Autodesk Inventor part; units mm, degrees
(part 2 of 3)
sketch "Sketch13" plane through (0, 0, 3.5) normal (0, 0, 1) x (1, 0, 0)
  line L0 (21.3323, 13.0987) -> (21.3323, 4.2537) construction
  line L1 (21.3323, 4.2537) -> (17.835, 4.2537) construction
  line L2 (17.835, 4.2537) -> (17.835, 13.0987) construction
  line L3 (17.835, 13.0987) -> (21.3323, 13.0987) construction
  spline S0 degree 2 poles (20.9109, 12.1453) (20.8266, 12.1453) (20.6749, 12.2054) (20.6222, 12.2591) knots 0 0 0 1 2 2 2
  spline S1 degree 2 poles (20.6222, 12.2591) (20.5559, 12.3265) (20.4874, 12.5088) (20.4874, 12.6478) knots 0 0 0 1 2 2 2
  line L4 (20.4874, 12.6478) -> (20.4874, 12.7943)
  line L5 (20.4874, 12.7943) -> (20.0028, 12.7943)
  line L6 (20.0028, 12.7943) -> (20.0028, 12.967)
  line L7 (20.0028, 12.967) -> (21.3028, 12.967)
  line L8 (21.3028, 12.967) -> (21.3028, 12.6405)
  spline S2 degree 2 poles (21.3028, 12.6405) (21.3028, 12.5246) (21.2649, 12.3623) (21.2217, 12.3002) knots 0 0 0 1 2 2 2
  spline S3 degree 2 poles (21.2217, 12.3002) (21.1722, 12.2275) (21.0194, 12.1453) (20.9109, 12.1453) knots 0 0 0 1 2 2 2
  spline S4 degree 2 poles (20.9056, 12.3255) (20.9731, 12.3255) (21.0721, 12.3718) (21.1037, 12.4192) knots 0 0 0 1 2 2 2
  spline S5 degree 2 poles (21.1037, 12.4192) (21.1311, 12.4603) (21.1532, 12.5699) (21.1532, 12.651) knots 0 0 0 1 2 2 2
  line L9 (21.1532, 12.651) -> (21.1532, 12.7943)
  line L10 (21.1532, 12.7943) -> (20.6349, 12.7943)
  line L11 (20.6349, 12.7943) -> (20.6349, 12.6763)
  spline S6 degree 2 poles (20.6349, 12.6763) (20.6349, 12.5709) (20.6686, 12.4414) (20.7128, 12.3992) knots 0 0 0 1 2 2 2
  spline S7 degree 2 poles (20.7128, 12.3992) (20.7518, 12.3602) (20.8435, 12.3255) (20.9056, 12.3255) knots 0 0 0 1 2 2 2
  spline S8 degree 2 poles (19.9796, 11.4732) (19.9796, 11.5996) (20.0649, 11.8135) (20.1503, 11.8914) knots 0 0 0 1 2 2 2
  spline S9 degree 2 poles (20.1503, 11.8914) (20.2346, 11.9694) (20.4874, 12.0547) (20.6517, 12.0547) knots 0 0 0 1 2 2 2
  spline S10 degree 2 poles (20.6517, 12.0547) (20.815, 12.0547) (21.0573, 11.9715) (21.1469, 11.8925) knots 0 0 0 1 2 2 2
  spline S11 degree 2 poles (21.1469, 11.8925) (21.2343, 11.8145) (21.326, 11.6017) (21.326, 11.47) knots 0 0 0 1 2 2 2
  spline S12 degree 2 poles (21.326, 11.47) (21.326, 11.4047) (21.307, 11.2899) (21.2923, 11.2414) knots 0 0 0 1 2 2 2
  spline S13 degree 2 poles (21.2923, 11.2414) (21.2786, 11.1993) (21.2396, 11.1119) (21.2164, 11.0687) knots 0 0 0 1 2 2 2
  line L12 (21.2164, 11.0687) -> (21.0078, 11.0687)
  line L13 (21.0078, 11.0687) -> (21.0078, 11.0824)
  spline S14 degree 2 poles (21.0078, 11.0824) (21.0289, 11.1055) (21.0879, 11.1772) (21.1163, 11.2288) knots 0 0 0 1 2 2 2
  spline S15 degree 2 poles (21.1163, 11.2288) (21.1437, 11.2783) (21.1785, 11.3952) (21.1785, 11.4711) knots 0 0 0 1 2 2 2
  spline S16 degree 2 poles (21.1785, 11.4711) (21.1785, 11.5543) (21.11, 11.7029) (21.0447, 11.7587) knots 0 0 0 1 2 2 2
  spline S17 degree 2 poles (21.0447, 11.7587) (20.9783, 11.8135) (20.7771, 11.8746) (20.6517, 11.8746) knots 0 0 0 1 2 2 2
  spline S18 degree 2 poles (20.6517, 11.8746) (20.5179, 11.8746) (20.3252, 11.8103) (20.2588, 11.7545) knots 0 0 0 1 2 2 2
  spline S19 degree 2 poles (20.2588, 11.7545) (20.1945, 11.6997) (20.1292, 11.5533) (20.1292, 11.4711) knots 0 0 0 1 2 2 2
  spline S20 degree 2 poles (20.1292, 11.4711) (20.1292, 11.3963) (20.1661, 11.2688) (20.1935, 11.2193) knots 0 0 0 1 2 2 2
  spline S21 degree 2 poles (20.1935, 11.2193) (20.2209, 11.1719) (20.2778, 11.1013) (20.2978, 11.0813) knots 0 0 0 1 2 2 2
  line L14 (20.2978, 11.0813) -> (20.2978, 11.0687)
  line L15 (20.2978, 11.0687) -> (20.0913, 11.0687)
  spline S22 degree 2 poles (20.0913, 11.0687) (20.0713, 11.1119) (20.0344, 11.1877) (20.0175, 11.2414) knots 0 0 0 1 2 2 2
  spline S23 degree 2 poles (20.0175, 11.2414) (19.9986, 11.2983) (19.9796, 11.3952) (19.9796, 11.4732) knots 0 0 0 1 2 2 2
  line L16 (21.149, 10.13) -> (21.149, 10.7347)
  line L17 (21.149, 10.7347) -> (20.7824, 10.7347)
  line L18 (20.7824, 10.7347) -> (20.7824, 10.1553)
  line L19 (20.7824, 10.1553) -> (20.6286, 10.1553)
  line L20 (20.6286, 10.1553) -> (20.6286, 10.7347)
  line L21 (20.6286, 10.7347) -> (20.0028, 10.7347)
  line L22 (20.0028, 10.7347) -> (20.0028, 10.9075)
  line L23 (20.0028, 10.9075) -> (21.3028, 10.9075)
  line L24 (21.3028, 10.9075) -> (21.3028, 10.13)
  line L25 (21.3028, 10.13) -> (21.149, 10.13)
  spline S24 degree 2 poles (19.9733, 9.6191) (19.9733, 9.716) (20.0312, 9.8751) (20.085, 9.9309) knots 0 0 0 1 2 2 2
  spline S25 degree 2 poles (20.085, 9.9309) (20.1376, 9.9857) (20.2809, 10.0426) (20.362, 10.0426) knots 0 0 0 1 2 2 2
  spline S26 degree 2 poles (20.362, 10.0426) (20.4674, 10.0426) (20.6444, 9.9298) (20.697, 9.8224) knots 0 0 0 1 2 2 2
  line L26 (20.697, 9.8224) -> (20.7023, 9.8224)
  spline S27 degree 2 poles (20.7023, 9.8224) (20.7581, 9.9183) (20.8909, 10.011) (20.9899, 10.011) knots 0 0 0 1 2 2 2
  spline S28 degree 2 poles (20.9899, 10.011) (21.1363, 10.011) (21.3323, 9.7897) (21.3323, 9.6191) knots 0 0 0 1 2 2 2
  spline S29 degree 2 poles (21.3323, 9.6191) (21.3323, 9.4421) (21.1469, 9.2282) (21.0015, 9.2282) knots 0 0 0 1 2 2 2
  spline S30 degree 2 poles (21.0015, 9.2282) (20.9141, 9.2282) (20.7434, 9.3304) (20.6949, 9.4263) knots 0 0 0 1 2 2 2
  line L27 (20.6949, 9.4263) -> (20.6897, 9.4263)
  spline S31 degree 2 poles (20.6897, 9.4263) (20.637, 9.3125) (20.4853, 9.1956) (20.3652, 9.1956) knots 0 0 0 1 2 2 2
  spline S32 degree 2 poles (20.3652, 9.1956) (20.1987, 9.1956) (19.9733, 9.4379) (19.9733, 9.6191) knots 0 0 0 1 2 2 2
  spline S33 degree 2 poles (20.3483, 9.3747) (20.4284, 9.3747) (20.5232, 9.4379) (20.5717, 9.5274) knots 0 0 0 1 2 2 2
  spline S34 degree 2 poles (20.5717, 9.5274) (20.5885, 9.5569) (20.6275, 9.6559) (20.6528, 9.7181) knots 0 0 0 1 2 2 2
  spline S35 degree 2 poles (20.6528, 9.7181) (20.6054, 9.7897) (20.4642, 9.8666) (20.3747, 9.8666) knots 0 0 0 1 2 2 2
  spline S36 degree 2 poles (20.3747, 9.8666) (20.2567, 9.8666) (20.1029, 9.7244) (20.1029, 9.617) knots 0 0 0 1 2 2 2
  spline S37 degree 2 poles (20.1029, 9.617) (20.1029, 9.5074) (20.2346, 9.3747) (20.3483, 9.3747) knots 0 0 0 1 2 2 2
  spline S38 degree 2 poles (20.9994, 9.3989) (21.0868, 9.3989) (21.2038, 9.5158) (21.2038, 9.6201) knots 0 0 0 1 2 2 2
  spline S39 degree 2 poles (21.2038, 9.6201) (21.2038, 9.7149) (21.0995, 9.8361) (21.0099, 9.8361) knots 0 0 0 1 2 2 2
  spline S40 degree 2 poles (21.0099, 9.8361) (20.9457, 9.8361) (20.8561, 9.7739) (20.8203, 9.7118) knots 0 0 0 1 2 2 2
  spline S41 degree 2 poles (20.8203, 9.7118) (20.8055, 9.6854) (20.7539, 9.5738) (20.7392, 9.5285) knots 0 0 0 1 2 2 2
  spline S42 degree 2 poles (20.7392, 9.5285) (20.7971, 9.4526) (20.9204, 9.3989) (20.9994, 9.3989) knots 0 0 0 1 2 2 2
  spline S43 degree 2 poles (20.4158, 8.2485) (20.322, 8.2485) (20.1619, 8.3085) (20.1029, 8.3633) knots 0 0 0 1 2 2 2
  spline S44 degree 2 poles (20.1029, 8.3633) (20.0439, 8.4181) (19.9754, 8.5814) (19.9754, 8.6825) knots 0 0 0 1 2 2 2
  spline S45 degree 2 poles (19.9754, 8.6825) (19.9754, 8.7752) (20.0165, 8.9564) (20.0491, 9.0228) knots 0 0 0 1 2 2 2
  line L28 (20.0491, 9.0228) -> (20.2335, 9.0228)
  line L29 (20.2335, 9.0228) -> (20.2335, 9.0102)
  spline S46 degree 2 poles (20.2335, 9.0102) (20.2188, 8.9901) (20.1808, 8.9153) (20.164, 8.87) knots 0 0 0 1 2 2 2
  spline S47 degree 2 poles (20.164, 8.87) (20.1461, 8.8184) (20.1261, 8.7331) (20.1261, 8.6794) knots 0 0 0 1 2 2 2
  spline S48 degree 2 poles (20.1261, 8.6794) (20.1261, 8.6267) (20.164, 8.5277) (20.2051, 8.4918) knots 0 0 0 1 2 2 2
  spline S49 degree 2 poles (20.2051, 8.4918) (20.244, 8.4592) (20.3473, 8.4255) (20.4168, 8.4255) knots 0 0 0 1 2 2 2
  spline S50 degree 2 poles (20.4168, 8.4255) (20.4863, 8.4255) (20.5748, 8.4634) (20.6043, 8.4992) knots 0 0 0 1 2 2 2
  spline S51 degree 2 poles (20.6043, 8.4992) (20.637, 8.5361) (20.6644, 8.6457) (20.6644, 8.712) knots 0 0 0 1 2 2 2
  spline S52 degree 2 poles (20.6644, 8.712) (20.6644, 8.7837) (20.6423, 8.9259) (20.6328, 8.9691) knots 0 0 0 1 2 2 2
  line L30 (20.6328, 8.9691) -> (21.3028, 8.9691)
  line L31 (21.3028, 8.9691) -> (21.3028, 8.2559)
  line L32 (21.3028, 8.2559) -> (21.15, 8.2559)
  line L33 (21.15, 8.2559) -> (21.15, 8.8016)
  line L34 (21.15, 8.8016) -> (20.8034, 8.8016)
  spline S53 degree 2 poles (20.8034, 8.8016) (20.8077, 8.77) (20.8108, 8.7089) (20.8108, 8.6836) knots 0 0 0 1 2 2 2
  spline S54 degree 2 poles (20.8108, 8.6836) (20.8108, 8.5835) (20.7782, 8.4455) (20.7297, 8.3823) knots 0 0 0 1 2 2 2
  spline S55 degree 2 poles (20.7297, 8.3823) (20.6812, 8.318) (20.5337, 8.2485) (20.4158, 8.2485) knots 0 0 0 1 2 2 2
  line L35 (21.1079, 7.2445) -> (20.0028, 7.8071)
  line L36 (20.0028, 7.8071) -> (20.0028, 7.9925)
  line L37 (20.0028, 7.9925) -> (21.15, 7.3983)
  line L38 (21.15, 7.3983) -> (21.15, 8.0694)
  line L39 (21.15, 8.0694) -> (21.3028, 8.0694)
  line L40 (21.3028, 8.0694) -> (21.3028, 7.2445)
  line L41 (21.3028, 7.2445) -> (21.1079, 7.2445)
  line L42 (20.4495, 6.249) -> (20.4495, 6.4038)
  line L43 (20.4495, 6.4038) -> (20.0028, 6.4038)
  line L44 (20.0028, 6.4038) -> (20.0028, 6.5713)
  line L45 (20.0028, 6.5713) -> (20.4495, 6.5713)
  line L46 (20.4495, 6.5713) -> (20.4495, 7.1455)
  line L47 (20.4495, 7.1455) -> (20.6328, 7.1455)
  line L48 (20.6328, 7.1455) -> (21.3028, 6.564)
  line L49 (21.3028, 6.564) -> (21.3028, 6.4038)
  line L50 (21.3028, 6.4038) -> (20.5896, 6.4038)
  line L51 (20.5896, 6.4038) -> (20.5896, 6.249)
  line L52 (20.5896, 6.249) -> (20.4495, 6.249)
  line L53 (20.5896, 6.5713) -> (21.0974, 6.5713)
  line L54 (21.0974, 6.5713) -> (20.5896, 7.0085)
  line L55 (20.5896, 7.0085) -> (20.5896, 6.5713)
  line L56 (20.4495, 5.2734) -> (20.4495, 5.4283)
  line L57 (20.4495, 5.4283) -> (20.0028, 5.4283)
  line L58 (20.0028, 5.4283) -> (20.0028, 5.5958)
  line L59 (20.0028, 5.5958) -> (20.4495, 5.5958)
  line L60 (20.4495, 5.5958) -> (20.4495, 6.17)
  line L61 (20.4495, 6.17) -> (20.6328, 6.17)
  line L62 (20.6328, 6.17) -> (21.3028, 5.5884)
  line L63 (21.3028, 5.5884) -> (21.3028, 5.4283)
  line L64 (21.3028, 5.4283) -> (20.5896, 5.4283)
  line L65 (20.5896, 5.4283) -> (20.5896, 5.2734)
  line L66 (20.5896, 5.2734) -> (20.4495, 5.2734)
  line L67 (20.5896, 5.5958) -> (21.0974, 5.5958)
  line L68 (21.0974, 5.5958) -> (20.5896, 6.033)
  line L69 (20.5896, 6.033) -> (20.5896, 5.5958)
  line L70 (20.0028, 4.398) -> (20.0028, 5.0322)
  line L71 (20.0028, 5.0322) -> (20.1355, 5.0322)
  line L72 (20.1355, 5.0322) -> (20.1355, 4.7962)
  line L73 (20.1355, 4.7962) -> (21.0068, 4.7962)
  line L74 (21.0068, 4.7962) -> (21.0068, 5.0322)
  line L75 (21.0068, 5.0322) -> (21.1258, 5.0322)
  spline S56 degree 2 poles (21.1258, 5.0322) (21.1258, 4.8984) (21.2017, 4.772) (21.307, 4.7636) knots 0 0 0 1 2 2 2
  line L76 (21.307, 4.7636) -> (21.307, 4.6287)
  line L77 (21.307, 4.6287) -> (20.1355, 4.6287)
  line L78 (20.1355, 4.6287) -> (20.1355, 4.398)
  line L79 (20.1355, 4.398) -> (20.0028, 4.398)
  line L80 (17.8624, 12.0231) -> (17.8624, 12.1959)
  line L81 (17.8624, 12.1959) -> (18.4987, 12.1959)
  line L82 (18.4987, 12.1959) -> (18.4987, 12.7943)
  line L83 (18.4987, 12.7943) -> (17.8624, 12.7943)
  line L84 (17.8624, 12.7943) -> (17.8624, 12.967)
  line L85 (17.8624, 12.967) -> (19.1624, 12.967)
  line L86 (19.1624, 12.967) -> (19.1624, 12.7943)
  line L87 (19.1624, 12.7943) -> (18.6525, 12.7943)
  line L88 (18.6525, 12.7943) -> (18.6525, 12.1959)
  line L89 (18.6525, 12.1959) -> (19.1624, 12.1959)
  line L90 (19.1624, 12.1959) -> (19.1624, 12.0231)
  line L91 (19.1624, 12.0231) -> (17.8624, 12.0231)
  line L92 (17.8624, 11.0065) -> (17.8624, 11.7598)
  line L93 (17.8624, 11.7598) -> (19.1624, 11.7598)
  line L94 (19.1624, 11.7598) -> (19.1624, 11.587)
  line L95 (19.1624, 11.587) -> (18.0162, 11.587)
  line L96 (18.0162, 11.587) -> (18.0162, 11.0065)
  line L97 (18.0162, 11.0065) -> (17.8624, 11.0065)
  line L98 (19.0086, 10.0931) -> (19.0086, 10.6978)
  line L99 (19.0086, 10.6978) -> (18.642, 10.6978)
  line L100 (18.642, 10.6978) -> (18.642, 10.1184)
  line L101 (18.642, 10.1184) -> (18.4881, 10.1184)
  line L102 (18.4881, 10.1184) -> (18.4881, 10.6978)
  line L103 (18.4881, 10.6978) -> (17.8624, 10.6978)
  line L104 (17.8624, 10.6978) -> (17.8624, 10.8706)
  line L105 (17.8624, 10.8706) -> (19.1624, 10.8706)
  line L106 (19.1624, 10.8706) -> (19.1624, 10.0931)
  line L107 (19.1624, 10.0931) -> (19.0086, 10.0931)
  line L108 (17.8624, 7.4984) -> (17.8624, 8.3001)
  line L109 (17.8624, 8.3001) -> (18.0467, 8.3001)
  spline S57 degree 2 poles (18.0467, 8.3001) (18.1279, 8.2137) (18.2785, 8.0599) (18.3596, 7.9862) knots 0 0 0 1 2 2 2
  spline S58 degree 2 poles (18.3596, 7.9862) (18.5229, 7.8376) (18.7189, 7.7291) (18.8232, 7.7291) knots 0 0 0 1 2 2 2
  spline S59 degree 2 poles (18.8232, 7.7291) (18.8779, 7.7291) (18.9601, 7.7628) (18.9864, 7.7934) knots 0 0 0 1 2 2 2
  spline S60 degree 2 poles (18.9864, 7.7934) (19.0128, 7.8239) (19.0391, 7.904) (19.0391, 7.9525) knots 0 0 0 1 2 2 2
  spline S61 degree 2 poles (19.0391, 7.9525) (19.0391, 7.9988) (19.0159, 8.0936) (18.998, 8.1368) knots 0 0 0 1 2 2 2
  spline S62 degree 2 poles (18.998, 8.1368) (18.9833, 8.1737) (18.9411, 8.2422) (18.9264, 8.2632) knots 0 0 0 1 2 2 2
  line L110 (18.9264, 8.2632) -> (18.9264, 8.2727)
  line L111 (18.9264, 8.2727) -> (19.1118, 8.2727)
  spline S63 degree 2 poles (19.1118, 8.2727) (19.1381, 8.219) (19.1898, 8.0262) (19.1898, 7.9398) knots 0 0 0 1 2 2 2
  spline S64 degree 2 poles (19.1898, 7.9398) (19.1898, 7.7576) (18.997, 7.5521) (18.8326, 7.5521) knots 0 0 0 1 2 2 2
  spline S65 degree 2 poles (18.8326, 7.5521) (18.7557, 7.5521) (18.6272, 7.588) (18.5724, 7.6196) knots 0 0 0 1 2 2 2
  spline S66 degree 2 poles (18.5724, 7.6196) (18.5155, 7.6512) (18.4039, 7.7428) (18.3501, 7.7934) knots 0 0 0 1 2 2 2
  spline S67 degree 2 poles (18.3501, 7.7934) (18.2606, 7.8756) (18.0689, 8.0768) (18.013, 8.1368) knots 0 0 0 1 2 2 2
  line L112 (18.013, 8.1368) -> (18.013, 7.4984)
  line L113 (18.013, 7.4984) -> (17.8624, 7.4984)
  line L114 (17.8624, 6.5882) -> (17.8624, 7.2224)
  line L115 (17.8624, 7.2224) -> (17.9951, 7.2224)
  line L116 (17.9951, 7.2224) -> (17.9951, 6.9864)
  line L117 (17.9951, 6.9864) -> (18.8663, 6.9864)
  line L118 (18.8663, 6.9864) -> (18.8663, 7.2224)
  line L119 (18.8663, 7.2224) -> (18.9854, 7.2224)
  spline S68 degree 2 poles (18.9854, 7.2224) (18.9854, 7.0886) (19.0612, 6.9622) (19.1666, 6.9538) knots 0 0 0 1 2 2 2
  line L120 (19.1666, 6.9538) -> (19.1666, 6.8189)
  line L121 (19.1666, 6.8189) -> (17.9951, 6.8189)
  line L122 (17.9951, 6.8189) -> (17.9951, 6.5882)
  line L123 (17.9951, 6.5882) -> (17.8624, 6.5882)
  line L124 (17.8624, 6.4523) -> (19.1624, 6.014)
  line L125 (19.1624, 6.014) -> (19.1624, 5.8012)
  line L126 (19.1624, 5.8012) -> (17.8624, 5.363)
  line L127 (17.8624, 5.363) -> (17.8624, 5.5452)
  line L128 (17.8624, 5.5452) -> (18.2258, 5.6632)
  line L129 (18.2258, 5.6632) -> (18.2258, 6.1594)
  line L130 (18.2258, 6.1594) -> (17.8624, 6.2774)
  line L131 (17.8624, 6.2774) -> (17.8624, 6.4523)
  line L132 (18.3733, 5.7106) -> (18.9854, 5.9119)
  line L133 (18.9854, 5.9119) -> (18.3733, 6.112)
  line L134 (18.3733, 6.112) -> (18.3733, 5.7106)
  spline S69 degree 2 poles (18.5124, 4.4675) (18.1626, 4.4675) (17.835, 4.6709) (17.835, 4.8826) knots 0 0 0 1 2 2 2
  spline S70 degree 2 poles (17.835, 4.8826) (17.835, 5.0975) (18.1689, 5.2987) (18.5113, 5.2987) knots 0 0 0 1 2 2 2
  spline S71 degree 2 poles (18.5113, 5.2987) (18.8632, 5.2987) (19.1887, 5.0954) (19.1887, 4.8826) knots 0 0 0 1 2 2 2
  spline S72 degree 2 poles (19.1887, 4.8826) (19.1887, 4.6687) (18.8516, 4.4675) (18.5124, 4.4675) knots 0 0 0 1 2 2 2
  spline S73 degree 2 poles (18.1163, 4.6909) (18.1805, 4.6656) (18.3786, 4.6445) (18.5124, 4.6445) knots 0 0 0 1 2 2 2
  spline S74 degree 2 poles (18.5124, 4.6445) (18.6462, 4.6445) (18.8432, 4.6656) (18.9095, 4.6919) knots 0 0 0 1 2 2 2
  spline S75 degree 2 poles (18.9095, 4.6919) (18.9759, 4.7183) (19.0444, 4.8099) (19.0444, 4.8826) knots 0 0 0 1 2 2 2
  spline S76 degree 2 poles (19.0444, 4.8826) (19.0444, 4.9553) (18.9759, 5.0491) (18.9074, 5.0764) knots 0 0 0 1 2 2 2
  spline S77 degree 2 poles (18.9074, 5.0764) (18.8411, 5.1028) (18.6388, 5.1217) (18.5113, 5.1217) knots 0 0 0 1 2 2 2
  spline S78 degree 2 poles (18.5113, 5.1217) (18.3744, 5.1217) (18.1911, 5.1049) (18.1194, 5.0775) knots 0 0 0 1 2 2 2
  spline S79 degree 2 poles (18.1194, 5.0775) (18.052, 5.0522) (17.9793, 4.9585) (17.9793, 4.8826) knots 0 0 0 1 2 2 2
  spline S80 degree 2 poles (17.9793, 4.8826) (17.9793, 4.811) (18.0478, 4.7172) (18.1163, 4.6909) knots 0 0 0 1 2 2 2
  point P0 (0, 0)
  dimension "d53" = 38.1
  dimension "d54" = 0.65
  dimension "d55" = 0.65
  dimension "d56" = 0.65
  dimension "d57" = 0.65
  dimension "d58" = 2.54
  dimension "d59" = 2.54
  dimension "d60" = 2.54
  dimension "d61" = 2.54
  dimension "d62" = 2.54
  dimension "d63" = 2.54
  dimension "d64" = 2.54
  dimension "d65" = 2.54
  dimension "d66" = 2.54
  dimension "d67" = 2.54
  dimension "d68" = 2.54
  dimension "d69" = 2.54
  dimension "d70" = 2.54
  dimension "d71" = 2.54
  dimension "d100" = 1.95
  dimension "d101" = 1.95
  dimension "d102" = 1.5
  dimension "d103" = 1.5
  dimension "d104" = 19
  constraints: 2 other
extrude "Extrusion11" add sketch "Sketch13" along normal blind 0.1
sketch "Sketch15" plane through (23.35, 3.6, 1) normal (1, 0, 0) x (0, 0, -1)
  line L0 (-2, 0) -> (-2, 10.3) projected
  line L1 (0, 0) -> (-2, 0) projected
  line L2 (0, 10.3) -> (0, 0) projected
  line L3 (0, 10.3) -> (-2, 10.3) projected
  line L4 (0, 0) -> (-2, 0) projected
  line L5 (-1, 0) -> (-1, 10.3)
  line L6 (-2, 10.3) -> (-1, 10.3)
  line L7 (-2.5, 0.5) -> (-2, 0) projected
  line L8 (-2, 0) -> (-1, 0)
  line L9 (-2, 10.3) -> (-2, 0) projected
  line L10 (-1.5, 8.2889) -> (-1, 8.2889)
  line L11 (-1.5, 9.5445) -> (-1, 9.5445)
  line L12 (-1.25, 1.2556) -> (-1.25, 0.2556)
  line L13 (-1.25, 0.2556) -> (-1.75, 0.2556)
  line L14 (-1.75, 0.2556) -> (-1.75, 1.2556)
  line L15 (-1.75, 1.2556) -> (-1.25, 1.2556)
  line L16 (-1.25, 1.2556) -> (-1.75, 0.2556) construction
  line L17 (-1.25, 0.2556) -> (-1.75, 1.2556) construction
  line L18 (-1.25, 2.5111) -> (-1.25, 1.5111)
  line L19 (-1.25, 1.5111) -> (-1.75, 1.5111)
  line L20 (-1.75, 1.5111) -> (-1.75, 2.5111)
  line L21 (-1.75, 2.5111) -> (-1.25, 2.5111)
  line L22 (-1.25, 2.5111) -> (-1.75, 1.5111) construction
  line L23 (-1.25, 1.5111) -> (-1.75, 2.5111) construction
  line L24 (-1.25, 3.7667) -> (-1.25, 2.7667)
  line L25 (-1.25, 2.7667) -> (-1.75, 2.7667)
  line L26 (-1.75, 2.7667) -> (-1.75, 3.7667)
  line L27 (-1.75, 3.7667) -> (-1.25, 3.7667)
  line L28 (-1.25, 3.7667) -> (-1.75, 2.7667) construction
  line L29 (-1.25, 2.7667) -> (-1.75, 3.7667) construction
  line L30 (-1.25, 5.0222) -> (-1.25, 4.0222)
  line L31 (-1.25, 4.0222) -> (-1.75, 4.0222)
  line L32 (-1.75, 4.0222) -> (-1.75, 5.0222)
  line L33 (-1.75, 5.0222) -> (-1.25, 5.0222)
  line L34 (-1.25, 5.0222) -> (-1.75, 4.0222) construction
  line L35 (-1.25, 4.0222) -> (-1.75, 5.0222) construction
  line L36 (-1.25, 6.2778) -> (-1.25, 5.2778)
  line L37 (-1.25, 5.2778) -> (-1.75, 5.2778)
  line L38 (-1.75, 5.2778) -> (-1.75, 6.2778)
  line L39 (-1.75, 6.2778) -> (-1.25, 6.2778)
  line L40 (-1.25, 6.2778) -> (-1.75, 5.2778) construction
  line L41 (-1.25, 5.2778) -> (-1.75, 6.2778) construction
  line L42 (-1.25, 7.5334) -> (-1.25, 6.5334)
  line L43 (-1.25, 6.5334) -> (-1.75, 6.5334)
  line L44 (-1.75, 6.5334) -> (-1.75, 7.5334)
  line L45 (-1.75, 7.5334) -> (-1.25, 7.5334)
  line L46 (-1.25, 7.5334) -> (-1.75, 6.5334) construction
  line L47 (-1.25, 6.5334) -> (-1.75, 7.5334) construction
  line L48 (-1.25, 8.7889) -> (-1.25, 7.7889)
  line L49 (-1.25, 7.7889) -> (-1.75, 7.7889)
  line L50 (-1.75, 7.7889) -> (-1.75, 8.7889)
  line L51 (-1.75, 8.7889) -> (-1.25, 8.7889)
  line L52 (-1.25, 8.7889) -> (-1.75, 7.7889) construction
  line L53 (-1.25, 7.7889) -> (-1.75, 8.7889) construction
  line L54 (-1.25, 10.0445) -> (-1.25, 9.0445)
  line L55 (-1.25, 9.0445) -> (-1.75, 9.0445)
  line L56 (-1.75, 9.0445) -> (-1.75, 10.0445)
  line L57 (-1.75, 10.0445) -> (-1.25, 10.0445)
  line L58 (-1.25, 10.0445) -> (-1.75, 9.0445) construction
  line L59 (-1.25, 9.0445) -> (-1.75, 10.0445) construction
  point P0 (1, -3.6)
  dimension "d240" = 10.3
  dimension "d257" = 10.3
  dimension "d276" = 0.5
  dimension "d277" = 0.5
  dimension "d278" = 0.5
  dimension "d279" = 0.5
  dimension "d280" = 0.5
  dimension "d281" = 0.5
  dimension "d282" = 0.5
  dimension "d283" = 0.5
  constraints: 106 end point, 16 parallel, 8 perpendicular, 2 collinear, 2 horizontal, 2 midpoint
  measures "d240" distance between parallel lines of L3 L1
  measures "d257" distance of L5.start L5.end
  measures "d276" distance of L12.end L13.end
  measures "d277" distance of L19.start L19.end
  measures "d278" distance of L25.start L25.end
  measures "d279" distance of L31.start L31.end
  measures "d280" distance of L37.start L37.end
  measures "d281" distance of L43.start L43.end
  measures "d282" distance of L49.start L49.end
  measures "d283" distance of L55.start L55.end
sketch "Sketch17" plane through (16.15, 13.9, 1) normal (0, 1, 0) x (1, 0, 0)
  line L0 (7.2, -2) -> (0, -2) projected
  line L1 (7.2, 0) -> (7.2, -2) projected
  line L2 (7.2, -2) -> (7.2, 0)
  line L3 (7.2, -1) -> (7.2, -2)
  line L4 (7.2, -1.5) -> (7.45, -1.5)
  arc A0 (7.45, -1.5) -> (7.95, -1) centre (7.45, -1) ccw
  line L5 (-18.1, 0) -> (23.9, 0) projected
  line L6 (8.2, 0) -> (7.95, 0)
  arc A1 (8.45, -0.25) -> (7.95, -0.75) centre (8.45, -0.75) ccw
  line L7 (7.95, -0.75) -> (7.95, -1)
  line L8 (8.45, -0.25) -> (8.7, -0.25)
  point P0 (-16.15, 1)
  dimension "d308" = 0.25
  dimension "d309" = 0.25
  constraints: 12 end point, 4 point on circle, 2 centre point, 2 horizontal, 2 midpoint, 2 point on line, 2 vertical, 1 collinear
  measures "d308" distance of L8.start L8.end
  measures "d309" distance of L4.start L4.end
sweep "Sweep1" add profiles "Sketch15" path "Sketch17" path curves L4 A0 L7 A1 L8 contours L48 L49 L50 L51 | L54 L55 L56 L57 | L12 L13 L14 L15 | L18 L19 L20 L21 | L24 L25 L26 L27 | L30 L31 L32 L33 | L36 L37 L38 L39 | L42 L43 L44 L45
ref_plane "Work Plane1" through (19.75, 3.6, 1) normal (1, 0, 0) x (0, 0, -1)
mirror "Mirror1" about plane through (19.75, 3.6, 1) normal (1, 0, 0) of "Sweep1"
sketch "Sketch18" plane through (0, 0, 2) normal (0, 0, 1) x (1, 0, 0)
  line L0 (25.4246, 15.877) -> (25.4246, 14.777) projected
  line L1 (25.4246, 15.877) -> (23.8246, 15.877) projected
  line L2 (23.8246, 14.777) -> (23.8246, 15.877) projected
  line L3 (23.8246, 14.777) -> (25.4246, 14.777) projected
  line L4 (21.5559, 15.7398) -> (21.5559, 14.6398) projected
  line L5 (21.5559, 15.7398) -> (19.9559, 15.7398) projected
  line L6 (19.9559, 14.6398) -> (19.9559, 15.7398) projected
  line L7 (19.9559, 14.6398) -> (21.5559, 14.6398) projected
  line L8 (18.3957, 15.7376) -> (18.3957, 14.6376) projected
  line L9 (18.3957, 15.7376) -> (16.7957, 15.7376) projected
  line L10 (16.7957, 14.6376) -> (16.7957, 15.7376) projected
  line L11 (16.7957, 14.6376) -> (18.3957, 14.6376) projected
  line L12 (25.1922, 15.0759) -> (24.0666, 15.0759) construction
  line L13 (24.0666, 15.0759) -> (24.0666, 15.5865) construction
  line L14 (24.0666, 15.5865) -> (25.1922, 15.5865) construction
  line L15 (25.1922, 15.5865) -> (25.1922, 15.0759) construction
  line L16 (21.3235, 14.9388) -> (20.1979, 14.9388) construction
  line L17 (20.1979, 14.9388) -> (20.1979, 15.4493) construction
  line L18 (20.1979, 15.4493) -> (21.3235, 15.4493) construction
  line L19 (21.3235, 15.4493) -> (21.3235, 14.9388) construction
  line L20 (18.1633, 14.9366) -> (17.0377, 14.9366) construction
  line L21 (17.0377, 14.9366) -> (17.0377, 15.4471) construction
  line L22 (17.0377, 15.4471) -> (18.1633, 15.4471) construction
  line L23 (18.1633, 15.4471) -> (18.1633, 14.9366) construction
  line L24 (24.834, 15.4147) -> (24.8936, 15.4147)
  line L25 (24.8936, 15.4147) -> (24.8936, 15.5865)
  line L26 (24.8936, 15.5865) -> (24.958, 15.5865)
  line L27 (24.958, 15.5865) -> (24.958, 15.4147)
  line L28 (24.958, 15.4147) -> (25.1788, 15.4147)
  line L29 (25.1788, 15.4147) -> (25.1788, 15.3442)
  line L30 (25.1788, 15.3442) -> (24.9552, 15.0865)
  line L31 (24.9552, 15.0865) -> (24.8936, 15.0865)
  line L32 (24.8936, 15.0865) -> (24.8936, 15.3608)
  line L33 (24.8936, 15.3608) -> (24.834, 15.3608)
  line L34 (24.834, 15.3608) -> (24.834, 15.4147)
  line L35 (24.958, 15.3608) -> (24.958, 15.1655)
  line L36 (24.958, 15.1655) -> (25.1261, 15.3608)
  line L37 (25.1261, 15.3608) -> (24.958, 15.3608)
  line L38 (24.4665, 15.1614) -> (24.6829, 15.5865)
  line L39 (24.6829, 15.5865) -> (24.7542, 15.5865)
  line L40 (24.7542, 15.5865) -> (24.5257, 15.1452)
  line L41 (24.5257, 15.1452) -> (24.7838, 15.1452)
  line L42 (24.7838, 15.1452) -> (24.7838, 15.0865)
  line L43 (24.7838, 15.0865) -> (24.4665, 15.0865)
  line L44 (24.4665, 15.0865) -> (24.4665, 15.1614)
  line L45 (24.097, 15.5865) -> (24.4053, 15.5865)
  line L46 (24.4053, 15.5865) -> (24.4053, 15.5156)
  spline S0 degree 2 poles (24.4053, 15.5156) (24.3721, 15.4844) (24.3129, 15.4264) (24.2846, 15.3952) knots 0 0 0 1 2 2 2
  spline S1 degree 2 poles (24.2846, 15.3952) (24.2274, 15.3324) (24.1857, 15.2571) (24.1857, 15.2169) knots 0 0 0 1 2 2 2
  spline S2 degree 2 poles (24.1857, 15.2169) (24.1857, 15.1959) (24.1987, 15.1643) (24.2104, 15.1541) knots 0 0 0 1 2 2 2
  spline S3 degree 2 poles (24.2104, 15.1541) (24.2222, 15.144) (24.253, 15.1339) (24.2716, 15.1339) knots 0 0 0 1 2 2 2
  spline S4 degree 2 poles (24.2716, 15.1339) (24.2894, 15.1339) (24.3259, 15.1428) (24.3425, 15.1497) knots 0 0 0 1 2 2 2
  spline S5 degree 2 poles (24.3425, 15.1497) (24.3567, 15.1554) (24.383, 15.1716) (24.3911, 15.1772) knots 0 0 0 1 2 2 2
  line L47 (24.3911, 15.1772) -> (24.3948, 15.1772)
  line L48 (24.3948, 15.1772) -> (24.3948, 15.1059)
  spline S6 degree 2 poles (24.3948, 15.1059) (24.3741, 15.0958) (24.3, 15.0759) (24.2667, 15.0759) knots 0 0 0 1 2 2 2
  spline S7 degree 2 poles (24.2667, 15.0759) (24.1966, 15.0759) (24.1176, 15.1501) (24.1176, 15.2133) knots 0 0 0 1 2 2 2
  spline S8 degree 2 poles (24.1176, 15.2133) (24.1176, 15.2429) (24.1314, 15.2923) (24.1436, 15.3134) knots 0 0 0 1 2 2 2
  spline S9 degree 2 poles (24.1436, 15.3134) (24.1557, 15.3353) (24.191, 15.3782) (24.2104, 15.3989) knots 0 0 0 1 2 2 2
  spline S10 degree 2 poles (24.2104, 15.3989) (24.242, 15.4333) (24.3194, 15.5071) (24.3425, 15.5285) knots 0 0 0 1 2 2 2
  line L49 (24.3425, 15.5285) -> (24.097, 15.5285)
  line L50 (24.097, 15.5285) -> (24.097, 15.5865)
  line L51 (20.9653, 15.2775) -> (21.0249, 15.2775)
  line L52 (21.0249, 15.2775) -> (21.0249, 15.4493)
  line L53 (21.0249, 15.4493) -> (21.0893, 15.4493)
  line L54 (21.0893, 15.4493) -> (21.0893, 15.2775)
  line L55 (21.0893, 15.2775) -> (21.3101, 15.2775)
  line L56 (21.3101, 15.2775) -> (21.3101, 15.207)
  line L57 (21.3101, 15.207) -> (21.0865, 14.9493)
  line L58 (21.0865, 14.9493) -> (21.0249, 14.9493)
  line L59 (21.0249, 14.9493) -> (21.0249, 15.2236)
  line L60 (21.0249, 15.2236) -> (20.9653, 15.2236)
  line L61 (20.9653, 15.2236) -> (20.9653, 15.2775)
  line L62 (21.0893, 15.2236) -> (21.0893, 15.0283)
  line L63 (21.0893, 15.0283) -> (21.2574, 15.2236)
  line L64 (21.2574, 15.2236) -> (21.0893, 15.2236)
  line L65 (20.5978, 15.0243) -> (20.8142, 15.4493)
  line L66 (20.8142, 15.4493) -> (20.8855, 15.4493)
  line L67 (20.8855, 15.4493) -> (20.657, 15.0081)
  line L68 (20.657, 15.0081) -> (20.9151, 15.0081)
  line L69 (20.9151, 15.0081) -> (20.9151, 14.9493)
  line L70 (20.9151, 14.9493) -> (20.5978, 14.9493)
  line L71 (20.5978, 14.9493) -> (20.5978, 15.0243)
  line L72 (20.2283, 15.4493) -> (20.5366, 15.4493)
  line L73 (20.5366, 15.4493) -> (20.5366, 15.3784)
  spline S11 degree 2 poles (20.5366, 15.3784) (20.5034, 15.3472) (20.4442, 15.2893) (20.4159, 15.2581) knots 0 0 0 1 2 2 2
  spline S12 degree 2 poles (20.4159, 15.2581) (20.3587, 15.1953) (20.317, 15.1199) (20.317, 15.0798) knots 0 0 0 1 2 2 2
  spline S13 degree 2 poles (20.317, 15.0798) (20.317, 15.0587) (20.33, 15.0271) (20.3417, 15.017) knots 0 0 0 1 2 2 2
  spline S14 degree 2 poles (20.3417, 15.017) (20.3535, 15.0069) (20.3843, 14.9967) (20.4029, 14.9967) knots 0 0 0 1 2 2 2
  spline S15 degree 2 poles (20.4029, 14.9967) (20.4207, 14.9967) (20.4572, 15.0056) (20.4738, 15.0125) knots 0 0 0 1 2 2 2
  spline S16 degree 2 poles (20.4738, 15.0125) (20.488, 15.0182) (20.5143, 15.0344) (20.5224, 15.0401) knots 0 0 0 1 2 2 2
  line L74 (20.5224, 15.0401) -> (20.5261, 15.0401)
  line L75 (20.5261, 15.0401) -> (20.5261, 14.9688)
  spline S17 degree 2 poles (20.5261, 14.9688) (20.5054, 14.9586) (20.4313, 14.9388) (20.398, 14.9388) knots 0 0 0 1 2 2 2
  spline S18 degree 2 poles (20.398, 14.9388) (20.3279, 14.9388) (20.2489, 15.0129) (20.2489, 15.0761) knots 0 0 0 1 2 2 2
  spline S19 degree 2 poles (20.2489, 15.0761) (20.2489, 15.1057) (20.2627, 15.1552) (20.2749, 15.1762) knots 0 0 0 1 2 2 2
  spline S20 degree 2 poles (20.2749, 15.1762) (20.287, 15.1981) (20.3223, 15.2411) (20.3417, 15.2617) knots 0 0 0 1 2 2 2
  spline S21 degree 2 poles (20.3417, 15.2617) (20.3733, 15.2962) (20.4507, 15.3699) (20.4738, 15.3914) knots 0 0 0 1 2 2 2
  line L76 (20.4738, 15.3914) -> (20.2283, 15.3914)
  line L77 (20.2283, 15.3914) -> (20.2283, 15.4493)
  line L78 (17.8051, 15.2753) -> (17.8647, 15.2753)
  line L79 (17.8647, 15.2753) -> (17.8647, 15.4471)
  line L80 (17.8647, 15.4471) -> (17.9291, 15.4471)
  line L81 (17.9291, 15.4471) -> (17.9291, 15.2753)
  line L82 (17.9291, 15.2753) -> (18.1499, 15.2753)
  line L83 (18.1499, 15.2753) -> (18.1499, 15.2048)
  line L84 (18.1499, 15.2048) -> (17.9262, 14.9471)
  line L85 (17.9262, 14.9471) -> (17.8647, 14.9471)
  line L86 (17.8647, 14.9471) -> (17.8647, 15.2214)
  line L87 (17.8647, 15.2214) -> (17.8051, 15.2214)
  line L88 (17.8051, 15.2214) -> (17.8051, 15.2753)
  line L89 (17.9291, 15.2214) -> (17.9291, 15.0261)
  line L90 (17.9291, 15.0261) -> (18.0972, 15.2214)
  line L91 (18.0972, 15.2214) -> (17.9291, 15.2214)
  line L92 (17.4376, 15.0221) -> (17.654, 15.4471)
  line L93 (17.654, 15.4471) -> (17.7253, 15.4471)
  line L94 (17.7253, 15.4471) -> (17.4967, 15.0059)
  line L95 (17.4967, 15.0059) -> (17.7549, 15.0059)
  line L96 (17.7549, 15.0059) -> (17.7549, 14.9471)
  line L97 (17.7549, 14.9471) -> (17.4376, 14.9471)
  line L98 (17.4376, 14.9471) -> (17.4376, 15.0221)
  line L99 (17.0681, 15.4471) -> (17.3764, 15.4471)
  line L100 (17.3764, 15.4471) -> (17.3764, 15.3762)
  spline S22 degree 2 poles (17.3764, 15.3762) (17.3432, 15.345) (17.284, 15.2871) (17.2557, 15.2559) knots 0 0 0 1 2 2 2
  spline S23 degree 2 poles (17.2557, 15.2559) (17.1985, 15.1931) (17.1568, 15.1177) (17.1568, 15.0776) knots 0 0 0 1 2 2 2
  spline S24 degree 2 poles (17.1568, 15.0776) (17.1568, 15.0565) (17.1698, 15.0249) (17.1815, 15.0148) knots 0 0 0 1 2 2 2
  spline S25 degree 2 poles (17.1815, 15.0148) (17.1933, 15.0046) (17.2241, 14.9945) (17.2427, 14.9945) knots 0 0 0 1 2 2 2
  spline S26 degree 2 poles (17.2427, 14.9945) (17.2605, 14.9945) (17.297, 15.0034) (17.3136, 15.0103) knots 0 0 0 1 2 2 2
  spline S27 degree 2 poles (17.3136, 15.0103) (17.3278, 15.016) (17.3541, 15.0322) (17.3622, 15.0379) knots 0 0 0 1 2 2 2
  line L101 (17.3622, 15.0379) -> (17.3659, 15.0379)
  line L102 (17.3659, 15.0379) -> (17.3659, 14.9666)
  spline S28 degree 2 poles (17.3659, 14.9666) (17.3452, 14.9564) (17.2711, 14.9366) (17.2378, 14.9366) knots 0 0 0 1 2 2 2
  spline S29 degree 2 poles (17.2378, 14.9366) (17.1677, 14.9366) (17.0887, 15.0107) (17.0887, 15.0739) knots 0 0 0 1 2 2 2
  spline S30 degree 2 poles (17.0887, 15.0739) (17.0887, 15.1035) (17.1025, 15.1529) (17.1147, 15.174) knots 0 0 0 1 2 2 2
  spline S31 degree 2 poles (17.1147, 15.174) (17.1268, 15.1959) (17.1621, 15.2388) (17.1815, 15.2595) knots 0 0 0 1 2 2 2
  spline S32 degree 2 poles (17.1815, 15.2595) (17.2131, 15.294) (17.2905, 15.3677) (17.3136, 15.3892) knots 0 0 0 1 2 2 2
  line L103 (17.3136, 15.3892) -> (17.0681, 15.3892)
  line L104 (17.0681, 15.3892) -> (17.0681, 15.4471)
  point P0 (0, 0)
  dimension "d53" = 38.1
  dimension "d54" = 0.65
  dimension "d55" = 0.65
  dimension "d56" = 0.65
  dimension "d57" = 0.65
  dimension "d58" = 2.54
  dimension "d59" = 2.54
  dimension "d60" = 2.54
  dimension "d61" = 2.54
  dimension "d62" = 2.54
  dimension "d63" = 2.54
  dimension "d64" = 2.54
  dimension "d65" = 2.54
  dimension "d66" = 2.54
  dimension "d67" = 2.54
  dimension "d68" = 2.54
  dimension "d69" = 2.54
  dimension "d70" = 2.54
  dimension "d71" = 2.54
  dimension "d100" = 1.95
  dimension "d101" = 1.95
  dimension "d102" = 1.5
  dimension "d103" = 1.5
  dimension "d104" = 19
  constraints: 6 other
extrude "Extrusion12" add sketch "Sketch18" along normal blind 0.1 contours L24 L25 L26 L27 L28 L29 L30 L31 L32 L33 L34 | L38 L39 L40 L41 L42 L43 L44 | L45 L46 S0 S1 S2 S3 S4 S5 L47 L48 S6 S7 S8 S9 S10 L49 L50 | L51 L52 L53 L54 L55 L56 L57 L58 L59 L60 L61 | L65 L66 L67 L68 L69 L70 L71 | L72 L73 S11 S12 S13 S14 S15 S16 L74 L75 S17 S18 S19 S20 S21 L76 L77 | L78 L79 L80 L81 L82 L83 L84 L85 L86 L87 L88 | L92 L93 L94 L95 L96 L97 L98 | L99 L100 S22 S23 S24 S25 S26 S27 L101 L102 S28 S29 S30 S31 S32 L103 L104
sketch "Sketch19" plane through (0, 0, 2) normal (0, 0, 1) x (1, 0, 0)
  line L0 (28.2585, 12.9872) -> (29.3585, 12.9872) projected
  line L1 (28.2585, 12.9872) -> (28.2585, 11.3872) projected
  line L2 (29.3585, 11.3872) -> (28.2585, 11.3872) projected
  line L3 (29.3585, 11.3872) -> (29.3585, 12.9872) projected
  line L4 (31.1887, 11.3872) -> (30.0887, 11.3872) projected
  line L5 (31.1887, 11.3872) -> (31.1887, 12.9872) projected
  line L6 (30.0887, 12.9872) -> (31.1887, 12.9872) projected
  line L7 (30.0887, 12.9872) -> (30.0887, 11.3872) projected
  line L8 (31.8382, 12.9872) -> (32.9382, 12.9872) projected
  line L9 (31.8382, 12.9872) -> (31.8382, 11.3872) projected
  line L10 (32.9382, 11.3872) -> (31.8382, 11.3872) projected
  line L11 (32.9382, 11.3872) -> (32.9382, 12.9872) projected
  line L12 (28.495, 11.6041) -> (28.495, 13.8553) construction
  line L13 (28.495, 13.8553) -> (29.516, 13.8553) construction
  line L14 (29.516, 13.8553) -> (29.516, 11.6041) construction
  line L15 (29.516, 11.6041) -> (28.495, 11.6041) construction
  line L16 (30.3322, 11.6041) -> (30.3322, 13.8553) construction
  line L17 (30.3322, 13.8553) -> (31.3533, 13.8553) construction
  line L18 (31.3533, 13.8553) -> (31.3533, 11.6041) construction
  line L19 (31.3533, 11.6041) -> (30.3322, 11.6041) construction
  line L20 (32.1266, 11.6413) -> (32.1266, 12.7669) construction
  line L21 (32.1266, 12.7669) -> (32.6476, 12.7669) construction
  line L22 (32.6476, 12.7669) -> (32.6476, 11.6413) construction
  line L23 (32.6476, 11.6413) -> (32.1266, 11.6413) construction
  line L24 (32.6371, 11.961) -> (32.6371, 11.7171)
  line L25 (32.6371, 11.7171) -> (32.586, 11.7171)
  line L26 (32.586, 11.7171) -> (32.586, 11.8078)
  line L27 (32.586, 11.8078) -> (32.2509, 11.8078)
  line L28 (32.2509, 11.8078) -> (32.2509, 11.7171)
  line L29 (32.2509, 11.7171) -> (32.2052, 11.7171)
  spline S0 degree 2 poles (32.2052, 11.7171) (32.2052, 11.7685) (32.176, 11.8171) (32.1355, 11.8204) knots 0 0 0 1 2 2 2
  line L30 (32.1355, 11.8204) -> (32.1355, 11.8722)
  line L31 (32.1355, 11.8722) -> (32.586, 11.8722)
  line L32 (32.586, 11.8722) -> (32.586, 11.961)
  line L33 (32.586, 11.961) -> (32.6371, 11.961)
  spline S1 degree 2 poles (32.3871, 12.3641) (32.5216, 12.3641) (32.6476, 12.2859) (32.6476, 12.2045) knots 0 0 0 1 2 2 2
  spline S2 degree 2 poles (32.6476, 12.2045) (32.6476, 12.1218) (32.5192, 12.0444) (32.3875, 12.0444) knots 0 0 0 1 2 2 2
  spline S3 degree 2 poles (32.3875, 12.0444) (32.2522, 12.0444) (32.127, 12.1226) (32.127, 12.2045) knots 0 0 0 1 2 2 2
  spline S4 degree 2 poles (32.127, 12.2045) (32.127, 12.2867) (32.2566, 12.3641) (32.3871, 12.3641) knots 0 0 0 1 2 2 2
  spline S5 degree 2 poles (32.5394, 12.2782) (32.5147, 12.288) (32.4385, 12.2961) (32.3871, 12.2961) knots 0 0 0 1 2 2 2
  spline S6 degree 2 poles (32.3871, 12.2961) (32.3356, 12.2961) (32.2599, 12.288) (32.2343, 12.2778) knots 0 0 0 1 2 2 2
  spline S7 degree 2 poles (32.2343, 12.2778) (32.2088, 12.2677) (32.1825, 12.2324) (32.1825, 12.2045) knots 0 0 0 1 2 2 2
  spline S8 degree 2 poles (32.1825, 12.2045) (32.1825, 12.1765) (32.2088, 12.1405) (32.2351, 12.1299) knots 0 0 0 1 2 2 2
  spline S9 degree 2 poles (32.2351, 12.1299) (32.2607, 12.1198) (32.3385, 12.1125) (32.3875, 12.1125) knots 0 0 0 1 2 2 2
  spline S10 degree 2 poles (32.3875, 12.1125) (32.4402, 12.1125) (32.5107, 12.119) (32.5382, 12.1295) knots 0 0 0 1 2 2 2
  spline S11 degree 2 poles (32.5382, 12.1295) (32.5642, 12.1393) (32.5921, 12.1753) (32.5921, 12.2045) knots 0 0 0 1 2 2 2
  spline S12 degree 2 poles (32.5921, 12.2045) (32.5921, 12.232) (32.5658, 12.2681) (32.5394, 12.2782) knots 0 0 0 1 2 2 2
  line L34 (32.6371, 12.7365) -> (32.6371, 12.4282)
  line L35 (32.6371, 12.4282) -> (32.5662, 12.4282)
  spline S13 degree 2 poles (32.5662, 12.4282) (32.535, 12.4614) (32.477, 12.5205) (32.4458, 12.5489) knots 0 0 0 1 2 2 2
  spline S14 degree 2 poles (32.4458, 12.5489) (32.383, 12.606) (32.3077, 12.6478) (32.2676, 12.6478) knots 0 0 0 1 2 2 2
  spline S15 degree 2 poles (32.2676, 12.6478) (32.2465, 12.6478) (32.2149, 12.6348) (32.2048, 12.623) knots 0 0 0 1 2 2 2
  spline S16 degree 2 poles (32.2048, 12.623) (32.1946, 12.6113) (32.1845, 12.5805) (32.1845, 12.5619) knots 0 0 0 1 2 2 2
  spline S17 degree 2 poles (32.1845, 12.5619) (32.1845, 12.544) (32.1934, 12.5076) (32.2003, 12.491) knots 0 0 0 1 2 2 2
  spline S18 degree 2 poles (32.2003, 12.491) (32.206, 12.4768) (32.2222, 12.4504) (32.2279, 12.4423) knots 0 0 0 1 2 2 2
  line L36 (32.2279, 12.4423) -> (32.2279, 12.4387)
  line L37 (32.2279, 12.4387) -> (32.1565, 12.4387)
  spline S19 degree 2 poles (32.1565, 12.4387) (32.1464, 12.4594) (32.1266, 12.5335) (32.1266, 12.5667) knots 0 0 0 1 2 2 2
  spline S20 degree 2 poles (32.1266, 12.5667) (32.1266, 12.6368) (32.2007, 12.7158) (32.2639, 12.7158) knots 0 0 0 1 2 2 2
  spline S21 degree 2 poles (32.2639, 12.7158) (32.2935, 12.7158) (32.3429, 12.7021) (32.364, 12.6899) knots 0 0 0 1 2 2 2
  spline S22 degree 2 poles (32.364, 12.6899) (32.3859, 12.6777) (32.4288, 12.6425) (32.4495, 12.623) knots 0 0 0 1 2 2 2
  spline S23 degree 2 poles (32.4495, 12.623) (32.4839, 12.5914) (32.5577, 12.5141) (32.5791, 12.491) knots 0 0 0 1 2 2 2
  line L38 (32.5791, 12.491) -> (32.5791, 12.7365)
  line L39 (32.5791, 12.7365) -> (32.6371, 12.7365)
  line L40 (30.6709, 11.9622) -> (30.6709, 11.9027)
  line L41 (30.6709, 11.9027) -> (30.8427, 11.9027)
  line L42 (30.8427, 11.9027) -> (30.8427, 11.8383)
  line L43 (30.8427, 11.8383) -> (30.6709, 11.8383)
  line L44 (30.6709, 11.8383) -> (30.6709, 11.6174)
  line L45 (30.6709, 11.6174) -> (30.6004, 11.6174)
  line L46 (30.6004, 11.6174) -> (30.3427, 11.8411)
  line L47 (30.3427, 11.8411) -> (30.3427, 11.9027)
  line L48 (30.3427, 11.9027) -> (30.617, 11.9027)
  line L49 (30.617, 11.9027) -> (30.617, 11.9622)
  line L50 (30.617, 11.9622) -> (30.6709, 11.9622)
  line L51 (30.617, 11.8383) -> (30.4217, 11.8383)
  line L52 (30.4217, 11.8383) -> (30.617, 11.6701)
  line L53 (30.617, 11.6701) -> (30.617, 11.8383)
  line L54 (30.4177, 12.3297) -> (30.8427, 12.1134)
  line L55 (30.8427, 12.1134) -> (30.8427, 12.0421)
  line L56 (30.8427, 12.0421) -> (30.4015, 12.2706)
  line L57 (30.4015, 12.2706) -> (30.4015, 12.0125)
  line L58 (30.4015, 12.0125) -> (30.3427, 12.0125)
  line L59 (30.3427, 12.0125) -> (30.3427, 12.3297)
  line L60 (30.3427, 12.3297) -> (30.4177, 12.3297)
  line L61 (30.8427, 12.6993) -> (30.8427, 12.3909)
  line L62 (30.8427, 12.3909) -> (30.7718, 12.3909)
  spline S24 degree 2 poles (30.7718, 12.3909) (30.7406, 12.4242) (30.6827, 12.4833) (30.6515, 12.5117) knots 0 0 0 1 2 2 2
  spline S25 degree 2 poles (30.6515, 12.5117) (30.5887, 12.5688) (30.5133, 12.6105) (30.4732, 12.6105) knots 0 0 0 1 2 2 2
  spline S26 degree 2 poles (30.4732, 12.6105) (30.4521, 12.6105) (30.4205, 12.5976) (30.4104, 12.5858) knots 0 0 0 1 2 2 2
  spline S27 degree 2 poles (30.4104, 12.5858) (30.4003, 12.5741) (30.3901, 12.5433) (30.3901, 12.5246) knots 0 0 0 1 2 2 2
  spline S28 degree 2 poles (30.3901, 12.5246) (30.3901, 12.5068) (30.3991, 12.4703) (30.4059, 12.4537) knots 0 0 0 1 2 2 2
  spline S29 degree 2 poles (30.4059, 12.4537) (30.4116, 12.4395) (30.4278, 12.4132) (30.4335, 12.4051) knots 0 0 0 1 2 2 2
  line L63 (30.4335, 12.4051) -> (30.4335, 12.4015)
  line L64 (30.4335, 12.4015) -> (30.3622, 12.4015)
  spline S30 degree 2 poles (30.3622, 12.4015) (30.3521, 12.4221) (30.3322, 12.4963) (30.3322, 12.5295) knots 0 0 0 1 2 2 2
  spline S31 degree 2 poles (30.3322, 12.5295) (30.3322, 12.5996) (30.4064, 12.6786) (30.4696, 12.6786) knots 0 0 0 1 2 2 2
  spline S32 degree 2 poles (30.4696, 12.6786) (30.4991, 12.6786) (30.5486, 12.6648) (30.5696, 12.6527) knots 0 0 0 1 2 2 2
  spline S33 degree 2 poles (30.5696, 12.6527) (30.5915, 12.6405) (30.6345, 12.6053) (30.6551, 12.5858) knots 0 0 0 1 2 2 2
  spline S34 degree 2 poles (30.6551, 12.5858) (30.6896, 12.5542) (30.7633, 12.4768) (30.7848, 12.4537) knots 0 0 0 1 2 2 2
  line L65 (30.7848, 12.4537) -> (30.7848, 12.6993)
  line L66 (30.7848, 12.6993) -> (30.8427, 12.6993)
  line L67 (28.8337, 11.9622) -> (28.8337, 11.9027)
  line L68 (28.8337, 11.9027) -> (29.0055, 11.9027)
  line L69 (29.0055, 11.9027) -> (29.0055, 11.8383)
  line L70 (29.0055, 11.8383) -> (28.8337, 11.8383)
  line L71 (28.8337, 11.8383) -> (28.8337, 11.6174)
  line L72 (28.8337, 11.6174) -> (28.7632, 11.6174)
  line L73 (28.7632, 11.6174) -> (28.5055, 11.8411)
  line L74 (28.5055, 11.8411) -> (28.5055, 11.9027)
  line L75 (28.5055, 11.9027) -> (28.7798, 11.9027)
  line L76 (28.7798, 11.9027) -> (28.7798, 11.9622)
  line L77 (28.7798, 11.9622) -> (28.8337, 11.9622)
  line L78 (28.7798, 11.8383) -> (28.5845, 11.8383)
  line L79 (28.5845, 11.8383) -> (28.7798, 11.6701)
  line L80 (28.7798, 11.6701) -> (28.7798, 11.8383)
  line L81 (28.5805, 12.3297) -> (29.0055, 12.1134)
  line L82 (29.0055, 12.1134) -> (29.0055, 12.0421)
  line L83 (29.0055, 12.0421) -> (28.5642, 12.2706)
  line L84 (28.5642, 12.2706) -> (28.5642, 12.0125)
  line L85 (28.5642, 12.0125) -> (28.5055, 12.0125)
  line L86 (28.5055, 12.0125) -> (28.5055, 12.3297)
  line L87 (28.5055, 12.3297) -> (28.5805, 12.3297)
  line L88 (29.0055, 12.6993) -> (29.0055, 12.3909)
  line L89 (29.0055, 12.3909) -> (28.9346, 12.3909)
  spline S35 degree 2 poles (28.9346, 12.3909) (28.9034, 12.4242) (28.8454, 12.4833) (28.8142, 12.5117) knots 0 0 0 1 2 2 2
  spline S36 degree 2 poles (28.8142, 12.5117) (28.7514, 12.5688) (28.6761, 12.6105) (28.636, 12.6105) knots 0 0 0 1 2 2 2
  spline S37 degree 2 poles (28.636, 12.6105) (28.6149, 12.6105) (28.5833, 12.5976) (28.5732, 12.5858) knots 0 0 0 1 2 2 2
  spline S38 degree 2 poles (28.5732, 12.5858) (28.563, 12.5741) (28.5529, 12.5433) (28.5529, 12.5246) knots 0 0 0 1 2 2 2
  spline S39 degree 2 poles (28.5529, 12.5246) (28.5529, 12.5068) (28.5618, 12.4703) (28.5687, 12.4537) knots 0 0 0 1 2 2 2
  spline S40 degree 2 poles (28.5687, 12.4537) (28.5744, 12.4395) (28.5906, 12.4132) (28.5963, 12.4051) knots 0 0 0 1 2 2 2
  line L90 (28.5963, 12.4051) -> (28.5963, 12.4015)
  line L91 (28.5963, 12.4015) -> (28.5249, 12.4015)
  spline S41 degree 2 poles (28.5249, 12.4015) (28.5148, 12.4221) (28.495, 12.4963) (28.495, 12.5295) knots 0 0 0 1 2 2 2
  spline S42 degree 2 poles (28.495, 12.5295) (28.495, 12.5996) (28.5691, 12.6786) (28.6323, 12.6786) knots 0 0 0 1 2 2 2
  spline S43 degree 2 poles (28.6323, 12.6786) (28.6619, 12.6786) (28.7113, 12.6648) (28.7324, 12.6527) knots 0 0 0 1 2 2 2
  spline S44 degree 2 poles (28.7324, 12.6527) (28.7543, 12.6405) (28.7972, 12.6053) (28.8179, 12.5858) knots 0 0 0 1 2 2 2
  spline S45 degree 2 poles (28.8179, 12.5858) (28.8523, 12.5542) (28.9261, 12.4768) (28.9476, 12.4537) knots 0 0 0 1 2 2 2
  line L92 (28.9476, 12.4537) -> (28.9476, 12.6993)
  line L93 (28.9476, 12.6993) -> (29.0055, 12.6993)
  point P0 (0, 0)
  dimension "d53" = 38.1
  dimension "d54" = 0.65
  dimension "d55" = 0.65
  dimension "d56" = 0.65
  dimension "d57" = 0.65
  dimension "d58" = 2.54
  dimension "d59" = 2.54
  dimension "d60" = 2.54
  dimension "d61" = 2.54
  dimension "d62" = 2.54
  dimension "d63" = 2.54
  dimension "d64" = 2.54
  dimension "d65" = 2.54
  dimension "d66" = 2.54
  dimension "d67" = 2.54
  dimension "d68" = 2.54
  dimension "d69" = 2.54
  dimension "d70" = 2.54
  dimension "d71" = 2.54
  dimension "d100" = 1.95
  dimension "d101" = 1.95
  dimension "d102" = 1.5
  dimension "d103" = 1.5
  dimension "d104" = 19
  constraints: 6 other
extrude "Extrusion13" add sketch "Sketch19" along normal blind 0.1 contours L24 L25 L26 L27 L28 L29 S0 L30 L31 L32 L33 | S1 S2 S3 S4 | L34 L35 S13 S14 S15 S16 S17 S18 L36 L37 S19 S20 S21 S22 S23 L38 L39 | L40 L41 L42 L43 L44 L45 L46 L47 L48 L49 L50 | L54 L55 L56 L57 L58 L59 L60 | L61 L62 S24 S25 S26 S27 S28 S29 L63 L64 S30 S31 S32 S33 S34 L65 L66 | L67 L68 L69 L70 L71 L72 L73 L74 L75 L76 L77 | L81 L82 L83 L84 L85 L86 L87 | L88 L89 S35 S36 S37 S38 S39 S40 L90 L91 S41 S42 S43 S44 S45 L92 L93